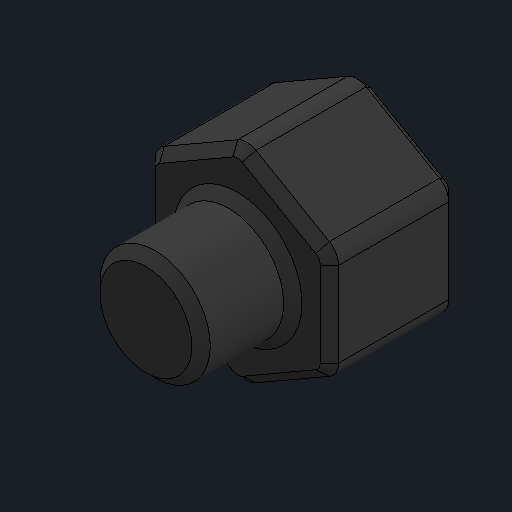
# Autodesk Inventor part: TPU-legs
Saved by Autodesk Inventor 2025 (Build 290162000, 162)
## iProperties
Created: 2024-05-30
Part Number: TPU-legs
Material: Rubber
Document SubType Name: Modeling
Designer: queezz
Density: 0.93 g/cm^3
Appearance: Rubber - Black
Author: queezz
Autodesk Inventor part; units mm, degrees
ref_plane "YZ Plane" through (0, 0, 0) normal (1, 0, 0) x (0, 1, 0)
ref_plane "XZ Plane" through (0, 0, 0) normal (0, 1, 0) x (-1, 0, 0)
ref_plane "XY Plane" through (0, 0, 0) normal (0, 0, 1) x (1, 0, 0)
sketch "Sketch1" plane through (0, 0, 0) normal (0, 0, 1) x (1, 0, 0)
  line L0 (5, 2.8868) -> (5, -2.8868)
  line L1 (5, -2.8868) -> (0, -5.7735)
  line L2 (0, -5.7735) -> (-5, -2.8868)
  line L3 (-5, -2.8868) -> (-5, 2.8868)
  line L4 (-5, 2.8868) -> (0, 5.7735)
  line L5 (0, 5.7735) -> (5, 2.8868)
  point P0 (0, 0)
  point P1 (0, 0)
  dimension "d0" = 10
  constraints: 12 end point, 1 coincident, 1 vertical, 13 other
  measures "d0" distance between parallel lines of L3 L0
extrude "Extrusion1" add sketch "Sketch1" along normal blind 7
sketch "Sketch2" plane through (0, 0, 7) normal (0, 0, 1) x (1, 0, 0)
  circle A0 centre (0, 0) radius 3
  dimension "d3" = 6
  constraints: 1 centre point, 1 coincident
  measures "d3" diameter of A0
extrude "Extrusion2" add sketch "Sketch2" along normal blind 5
fillet "Fillet1" radius 1 6 edges at (-5, 2.8868, 3.5) (-5, -2.8868, 3.5) (0, -5.7735, 3.5) (5, -2.8868, 3.5) (5, 2.8868, 3.5) (0, 5.7735, 3.5)
chamfer "Chamfer1" distance 0.5 angle 45 1 edges at (-3, 0, 7)
chamfer "Chamfer2" distance 0.5 angle 45 25 edges at (-3, 0, 12) (2.5, -4.3301, 7) (4.866, -2.8094, 7) (5, 0, 7) (4.866, 2.8094, 7) (2.5, 4.3301, 7) (0, 5.6188, 7) (-2.5, 4.3301, 7) (-4.866, 2.8094, 7) (-5, 0, 7) (-4.866, -2.8094, 7) (-2.5, -4.3301, 7) (0, -5.6188, 7) (2.5, -4.3301, 0) (4.866, -2.8094, 0) (5, 0, 0) (4.866, 2.8094, 0) (2.5, 4.3301, 0) (0, 5.6188, 0) (-2.5, 4.3301, 0) (-4.866, 2.8094, 0) (-5, 0, 0) (-4.866, -2.8094, 0) (-2.5, -4.3301, 0) (0, -5.6188, 0)
body "Solid1"
